pipe_join (Autodesk Fusion 360 design; units mm, degrees)
Autodesk Fusion 360 part; units mm, degrees
sketch "Sketch2" plane through (0, 0, 0) normal (0, 0, 1) x (1, 0, 0)
  line L0 (0, 0) -> (0, 65)
  line L1 (13.4496, 0.1022) -> (13.4496, 20.1022)
  line L2 (13.4496, 20.1022) -> (15.9496, 20.1022)
  line L3 (15.9496, 20.1022) -> (15.9496, 28.1022)
  line L4 (15.9496, 28.1022) -> (13.4496, 28.1022)
  line L5 (13.4496, 28.1022) -> (13.4496, 48.1022)
  line L6 (11.4496, 0.1022) -> (11.4496, 22.1022)
  line L7 (11.4496, 22.1022) -> (13.9496, 22.1022)
  line L8 (13.9496, 22.1022) -> (13.9496, 26.1022)
  line L9 (13.9496, 26.1022) -> (11.4496, 26.1022)
  line L10 (11.4496, 26.1022) -> (11.4496, 48.1022)
  line L11 (13.4496, 48.1022) -> (11.4496, 48.1022)
  line L12 (11.4496, 0.1022) -> (13.4496, 0.1022)
  line L13 (11.4496, 26.1022) -> (11.4496, 22.1022)
  line L14 (13.4496, 20.1022) -> (15.9496, 21.6691)
  line L15 (15.9496, 24.1022) -> (11.5, 24.1022)
  line L16 (13.4496, 28.1022) -> (15.9496, 26.5353)
  dimension "d2" = 13.45
  dimension "d3" = 20
  dimension "d4" = 20
  dimension "d5" = 8
  dimension "d6" = 2.5
  dimension "d7" = -2
  constraint coincident L0.start origin
  constraint vertical L0
  constraint parallel L0 L1
  constraint perpendicular L1 L2
  constraint perpendicular L2 L3
  constraint perpendicular L3 L4
  constraint perpendicular L4 L5
  constraint collinear L1 L5
  constraint perpendicular L5 L11
  constraint perpendicular L1 L12
  constraint coincident L3 L14.end
  constraint midpoint L3 L15.start
  constraint perpendicular L8 L15
  constraint symmetric L1.end L15 L4.end
  constraint symmetric L14.end L15 L16.end
  measures "d2" distance of L0.start L1.start
  measures "d3" distance of L1.start L1.end
  measures "d4" distance of L4.end L5.end
  measures "d5" distance of L2.end L3.end
  measures "d6" distance of L1.end L2.end
revolve "Revolve1" add sketch "Sketch2" angle 360 about axis through (0, 0, 0) along (0, 1, 0) contours L1 L3 L6 L7 L8 L12 L14 L15 | L7 L8 L9 L13 | L3 L5 L8 L9 L10 L11 L15 L16
equation "d2 = ( 26.9 / 2 ) * 1 mm"
equation "d4 = d3"
